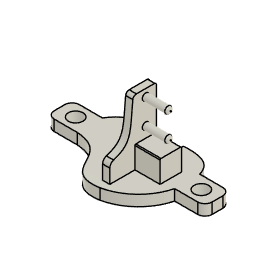
Uchyt na koncovy doraz (Autodesk Fusion 360 design; units mm, degrees)
Autodesk Fusion 360 part; units mm, degrees
note: some values were not read from the file. Set by a fixed rule: which sketch regions a step uses.
sketch "Sketch1" plane through (0, 0, 0) normal (0, 0, 1) x (1, 0, 0)
  line L0 (22, 1.5) -> (22, -1.5)
  line L1 (-22, -1.5) -> (-22, 1.5)
  circle A0 centre (-17.5, 0) radius 2.05
  circle A1 centre (17.5, 0) radius 2.05
  line L2 (-20, 3.5) -> (-13.5554, 3.5)
  line L3 (13.5554, 3.5) -> (20, 3.5)
  line L4 (20, -3.5) -> (13.5554, -3.5)
  line L5 (-13.5554, -3.5) -> (-20, -3.5)
  arc A2 (2.9858, -13.6779) -> (13.5554, -3.5) centre (0, 0) ccw
  arc A3 (22, 1.5) -> (20, 3.5) centre (20, 1.5) ccw
  arc A4 (20, -3.5) -> (22, -1.5) centre (20, -1.5) ccw
  arc A5 (-20, 3.5) -> (-22, 1.5) centre (-20, 1.5) ccw
  arc A6 (-22, -1.5) -> (-20, -3.5) centre (-20, -1.5) ccw
  circle A7 centre (0, 8) radius 4.55
  circle A8 centre (0, 8) radius 2.5
  spline S0 degree 5 poles (-13.5554, 3.5) (-13.4403, 3.6899) (-13.2044, 4.0607) (-12.8333, 4.5904) (-12.3036, 5.2425) (-11.5792, 5.9613) (-10.7872, 6.5756) (-9.9224, 7.0772) (-8.9826, 7.4626) (-7.9714, 7.7375) (-6.8944, 7.9106) (-5.9846, 7.9745) (-5.2769, 7.9832) (-4.794, 7.9718) (-4.5498, 7.9619) knots 0 0 0 0 0 0 0.1 0.2 0.3 0.4 0.5 0.6 0.7 0.8 0.9 1 1 1 1 1 1
  spline S1 degree 5 poles (13.5554, 3.5) (13.4982, 3.7035) (13.3727, 4.1002) (13.1508, 4.664) (12.7869, 5.3525) (12.2112, 6.1007) (11.5055, 6.7281) (10.6616, 7.2269) (9.6796, 7.5974) (8.5689, 7.8482) (7.3412, 7.9903) (6.2741, 8.0248) (5.429, 8.0092) (4.8462, 7.9807) (4.5498, 7.9619) knots 0 0 0 0 0 0 0.1 0.2 0.3 0.4 0.5 0.6 0.7 0.8 0.9 1 1 1 1 1 1
  spline S2 degree 5 poles (-13.5554, -3.5) (-13.2832, -3.5207) (-12.7507, -3.5722) (-11.9881, -3.6799) (-11.0436, -3.8844) (-9.9844, -4.2425) (-9.0464, -4.7029) (-8.2259, -5.2635) (-7.5154, -5.9188) (-6.9, -6.6582) (-6.3595, -7.4662) (-5.8692, -8.3231) (-5.4024, -9.2053) (-4.9312, -10.086) (-4.4284, -10.9351) (-3.8687, -11.7217) (-3.2294, -12.4165) (-2.4919, -12.994) (-1.6428, -13.4356) (-0.6752, -13.7313) (0.4139, -13.8766) (1.3823, -13.872) (2.163, -13.8011) (2.7075, -13.724) (2.9858, -13.6779) knots 0 0 0 0 0 0 0.05 0.1 0.15 0.2 0.25 0.3 0.35 0.4 0.45 0.5 0.55 0.6 0.65 0.7 0.75 0.8 0.85 0.9 0.95 1 1 1 1 1 1
  point P0 (-22, 3.5)
  point P1 (22, 3.5)
  point P2 (-22, -3.5)
  point P3 (-10, 7)
  point P4 (11, 7)
  point P5 (-8.024, -5.4772)
  point P6 (-5.3692, -9.2647)
  point P7 (-2.6437, -12.8398)
  dimension "d1" = 44
  dimension "d2" = 28
  dimension "d3" = 7
  dimension "d4" = 3.5
  dimension "d5" = 22
  dimension "d6" = 4.1
  dimension "d7" = 17.5
  dimension "d8" = 4.1
  dimension "d9" = 17.5
  dimension "d10" = 2
  dimension "d11" = 9.1
  dimension "d12" = 8
  dimension "d38" = 5
  constraint coincident A2.centre origin
  constraint horizontal L2
  constraint vertical L0
  constraint horizontal L4
  constraint vertical L1
  constraint coincident L3.start A2
  constraint collinear L2 L3
  constraint coincident L5.start L4
  constraint collinear L4 L5
  constraint coincident P1 L0
  constraint coincident P1 L3
  constraint tangent L0 A3
  constraint tangent L3 A3
  constraint tangent L0 A4
  constraint tangent L4 A4
  constraint equal A3 A4
  constraint coincident P0 L1
  constraint coincident P0 L2
  constraint tangent L1 A5
  constraint tangent L2 A5
  constraint equal A3 A5
  constraint coincident P2 L1
  constraint coincident P2 L5
  constraint tangent L1 A6
  constraint tangent L5 A6
  constraint equal A3 A6
  constraint concentric A7 A8
  constraint coincident A7 S0.end
  constraint coincident A7 S1.end
  measures "d1" distance of P0 P1
  measures "d2" diameter of A2
  measures "d3" distance of P0 P2
  measures "d4" distance of A2.centre L2
  measures "d5" distance of A2.centre L1
  measures "d6" diameter of A0
  measures "d7" distance of A2.centre A0.centre
  measures "d8" diameter of A1
  measures "d9" distance of A2.centre A1.centre
  measures "d10" radius of A3
  measures "d11" diameter of A7
  measures "d12" distance of A2.centre A7.centre
  measures "d38" diameter of A8
extrude "Extrude1" add sketch "Sketch1" along normal blind 2 contours L0 L1 L2 L3 L4 L5 A2 A3 A4 A5 A6 A7 S0 S1 S2
ref_plane "WorkPlane2" through (2.5, 0, 12.125) normal (1, 0, 0) x (0, 0, 1)
sketch "Sketch3" plane through (2.5, 0, 12.125) normal (1, 0, 0) x (0, 1, 0)
  line L0 (-4.0924, 9) -> (1.5, 9)
  line L1 (1.5, 9) -> (1.5, -11)
  line L2 (1.5, -11) -> (-11.5, -11)
  line L3 (-11.5, -11) -> (-11.5, -5.1958)
  circle A0 centre (-1.5, 7) radius 0.95
  circle A1 centre (-1.5, 0) radius 0.95
  line L4 (-4.5, -3) -> (1.5, -3)
  line L5 (1.5, -3) -> (1.5, -11)
  line L6 (1.5, -11) -> (-4.5, -11)
  line L7 (-4.5, -11) -> (-4.5, -3)
  spline S0 degree 5 poles (-10.4562, -3.7668) (-10.2158, -3.6901) (-9.7455, -3.5307) (-9.072, -3.2741) (-8.2432, -2.8843) (-7.3521, -2.2495) (-6.6362, -1.3928) (-6.1133, -0.2594) (-5.7654, 1.1445) (-5.5459, 2.7614) (-5.3974, 4.5131) (-5.29, 5.9577) (-5.1959, 7.0367) (-5.1246, 7.7503) (-5.0868, 8.1057) knots 0 0 0 0 0 0 0.1 0.2 0.3 0.4 0.5 0.6 0.7 0.8 0.9 1 1 1 1 1 1
  arc A2 (-4.0924, 9) -> (-5.0868, 8.1057) centre (-4.0924, 8) ccw
  arc A3 (-10.4562, -3.7668) -> (-11.5, -5.1958) centre (-10, -5.1958) ccw
  point P0 (-6.5, -1)
  dimension "d21" = 9
  dimension "d23" = 1.5
  dimension "d32" = 1.9
  dimension "d33" = 1.9
  dimension "d34" = 7
  dimension "d35" = 3
  dimension "d36" = 8
  dimension "d37" = 6
  dimension "d47" = 1
  dimension "d48" = 1.5
  dimension "d73" = 5.5924
  dimension "d74" = 13
  dimension "d75" = 10
  dimension "d88" = 2
  dimension "d89" = 3
  constraint horizontal L0
  constraint vertical L1
  constraint horizontal L2
  constraint vertical L3
  constraint horizontal L4
  constraint vertical L5
  constraint horizontal L6
  constraint vertical L7
  constraint tangent S0 A2
  constraint tangent L0 A2
  constraint tangent S0 A3
  constraint tangent L3 A3
  measures "d21" distance of origin L0
  measures "d23" distance of origin L1
  measures "d32" diameter of A0
  measures "d33" diameter of A1
  measures "d34" distance of A0.centre A1.centre
  measures "d35" distance of A1.centre L4
  measures "d36" distance of L4.start L6.end
  measures "d37" distance of L4.start L4.end
  measures "d47" radius of A2
  measures "d48" radius of A3
  measures "d73" distance of L0.end L0.start
  measures "d74" distance of L1.end L2.end
  measures "d75" distance of L3 A1.centre
  measures "d88" distance of L0 A0.centre
  measures "d89" distance of origin L4
extrude "Extrude12" add 1 faces at (-0.4768, -5.597, 2) along direction (0, 0, 1) blind 1
extrude "Extrude5" add sketch "Sketch3" along normal blind -1 and the other way blind -1 contours L0 L1 L2 L3 L4 L7 S0 A2 A3 | L1 L2 L4 L5 L6 L7 | A0 | A1
extrude "Extrude6" add sketch "Sketch3" along normal blind 8 contours L1 L2 L4 L5 L6 L7 | A0 | A1
fillet "Fillet1" radius 0.75 1 edges at (10.5, -2.3857, 11.7815)
fillet "Fillet2" radius 0.75 1 edges at (10.5, -2.3857, 18.7815)
fillet "Fillet4" radius 0.5 1 edges at (2.5, 1.5, 21.125)
fillet "Fillet3" radius 0.25 2 edges at (7, -4.5, 9.125) (7, 1.5, 9.125)
